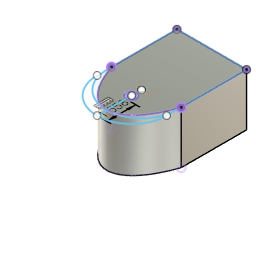
1759811952310_peo6bbk9y (Autodesk Fusion 360 archive; units mm, degrees)
design "dado_v3"
part number: 2025-08-25-22-53-08-385
Autodesk Fusion 360 part; units mm, degrees
sketch "Sketch1" plane through (0, 0, 0) normal (0, 0, 1) x (1, 0, 0)
  circle A0 centre (0, 0) radius 50.8
  line L0 (-50.8, 0) -> (50.8, 0)
  line L1 (50.8, 0) -> (50.8, 102.3291)
  line L2 (50.8, 102.3291) -> (-50.8, 102.3291)
  line L3 (-50.8, 102.3291) -> (-50.8, 0)
  dimension "d1" = 101.6
  constraint coincident A0.centre origin
  constraint horizontal L0
  constraint vertical L1
  constraint horizontal L2
  constraint vertical L3
  constraint coincident A0 L0.start
  constraint tangent A0 L1
  constraint tangent A0 L3
  measures "d1" diameter of A0
extrude "Extrude1" add sketch "Sketch1" along normal blind 76.2
sketch "Sketch2" plane through (0, 0, 76.2) normal (0, 0, 1) x (-1, 0, 0)
  line L0 (50.8, -102.3291) -> (50.8, 0)
  arc A0 (50.8, 0) -> (-50.8, 0) centre (0, 0) ccw
  line L1 (-50.8, 0) -> (-50.8, -102.3291)
  line L2 (-50.8, -102.3291) -> (50.8, -102.3291)
  circle A1 centre (-29.5656, 14.9606) radius 6.731
  circle A2 centre (-29.5656, -10.4394) radius 6.731
  circle A3 centre (-29.5656, -35.8394) radius 6.731
  circle A4 centre (29.5656, -35.8394) radius 6.731
  circle A5 centre (29.5656, -10.4394) radius 6.731
  circle A6 centre (29.5656, 14.9606) radius 6.731
  circle A7 centre (0, 14.9606) radius 7.874
  circle A8 centre (0, -35.8394) radius 7.874
  line L3 (0, 50.8) -> (0, 22.8346)
  line L4 (0, 14.9606) -> (-29.5656, 14.9606)
  line L5 (0, 14.9606) -> (29.5656, 14.9606)
  line L6 (-29.5656, -35.8394) -> (29.5656, -35.8394)
  line L7 (0, -35.8394) -> (0, -63.8048)
  dimension "d4" = 13.462
  dimension "d10" = 15.748
  dimension "d11" = 25.4
  dimension "d12" = 25.4
  dimension "d13" = 25.4
  dimension "d14" = 25.4
  dimension "d15" = 21.2344
  dimension "d16" = 21.2344
  dimension "d17" = 21.2344
  dimension "d18" = 21.2344
  dimension "d19" = 21.2344
  dimension "d20" = 21.2344
  dimension "d21" = 27.9654
  dimension "d22" = 27.9654
  constraint equal A1 A2
  constraint equal A1 A3
  constraint equal A1 A6
  constraint equal A1 A5
  constraint equal A1 A4
  constraint equal A7 A8
  constraint midpoint A0 L3.start
  constraint coincident A7 L3.end
  constraint vertical L3
  constraint coincident A7.centre L4.start
  constraint horizontal L4
  constraint coincident A1.centre L4.end
  constraint parallel L4 L5
  constraint coincident A6.centre L5.end
  constraint coincident A3.centre L6.start
  constraint coincident A4.centre L6.end
  constraint coincident A8.centre L6
  constraint coincident A8.centre L7.start
  constraint perpendicular L6 L7
  measures "d4" diameter of A1
  measures "d10" diameter of A7
  measures "d11" distance of A1.centre A2.centre
  measures "d12" distance of A2.centre A3.centre
  measures "d13" vertical distance of A5.centre A6.centre
  measures "d14" distance of A4.centre A5.centre
  measures "d15" distance of L1 A1.centre
  measures "d16" distance of L0 A6.centre
  measures "d17" distance of L1 A2.centre
  measures "d18" distance of L1 A3.centre
  measures "d19" distance of L0 A5.centre
  measures "d20" distance of L0 A4.centre
  measures "d21" distance of L3.start L3.end
  measures "d22" distance of A8.centre L7.end
extrude "Extrude2" cut sketch "Sketch2" against normal blind 101.6 contours A7 L4 L5 | A7 L4 L5
sketch "Sketch3" plane through (0, 0, 76.2) normal (0, 0, 1) x (-1, 0, 0)
  circle A0 centre (0, 14.9606) radius 7.874
  line L0 (50.8, -102.3291) -> (50.8, 0)
  arc A1 (50.8, 0) -> (-50.8, 0) centre (0, 0) ccw
  line L1 (-50.8, 0) -> (-50.8, -102.3291)
  line L2 (-50.8, -102.3291) -> (50.8, -102.3291)
  line L3 (-44.45, 12.7) -> (44.45, 12.7)
  line L4 (44.45, 12.7) -> (44.45, -102.3291)
  line L5 (44.45, -102.3291) -> (-44.45, -102.3291)
  line L6 (-44.45, -102.3291) -> (-44.45, 12.7)
  line L7 (0, 50.8) -> (0, 12.7)
  line L8 (0, 12.7) -> (0, 185.42)
  line L9 (-62.23, -56.8043) -> (62.23, -56.8043)
  spline S0 degree 2 poles (-62.23, -56.8043) (0, 395.5384) (62.23, -56.8043) knots 0 0 0 24.849245 24.849245 24.849245 weights 1 0.311883 1
  line L10 (-44.45, 9.235) -> (0, 9.235)
  line L11 (0, 50.8) -> (50.8, 50.8)
  line L12 (50.8, 50.8) -> (50.8, 0)
  line L13 (50.8, 0) -> (0, 0)
  line L14 (0, 0) -> (0, 50.8)
  line L15 (-43.815, 12.7) -> (43.815, 12.7)
  spline S1 degree 2 poles (43.815, 12.7) (0, 129.3943) (-43.815, 12.7) knots 0 0 0 12.094999 12.094999 12.094999 weights 1 0.555689 1
  line L16 (0, 12.7) -> (0, 17.78)
  dimension "d25" = 88.9
  dimension "d26" = 101.6
  dimension "d27" = 6.35
  dimension "d28" = 38.1
  dimension "d35" = 124.46
  dimension "d36" = 62.23
  dimension "d39" = 50.8
  constraint horizontal L3
  constraint vertical L4
  constraint horizontal L5
  constraint vertical L6
  constraint coincident L2 L4.end
  constraint midpoint A1 L7.start
  constraint perpendicular L3 L7
  constraint coincident L3 L7.end
  constraint perpendicular L3 L8
  constraint perpendicular L0 L9
  constraint coincident S0 L10.start
  constraint coincident L6 L10.start
  constraint perpendicular L6 L10
  constraint horizontal L11
  constraint vertical L12
  constraint horizontal L13
  constraint vertical L14
  constraint collinear L3 L15
  constraint midpoint L15 L7.end
  constraint perpendicular L15 L16
  constraint collinear L7 L16
  measures "d25" distance of L3.start L3.end
  measures "d26" distance of L0.start L1.end
  measures "d27" distance of L1 L6
  measures "d28" distance of L7.start L7.end
  measures "d35" distance of L9.start L9.end
  measures "d36" horizontal distance of L7.end L9.start
  measures "d39" distance of L7.start A1.centre
extrude "Extrude3" cut sketch "Sketch3" against normal blind 76.2 contours A1 L3 L7 L8 S0 L14 L15 S1 | A1 L3 L7 L8 S0 L14 L15 S1 | L3 L4 S0 L15 | L3 L6 S0 L15 | A1 L11 S1 | A1 L3 L4 S0 L13 S1 | A1 L1 L3 L6 S0 S1 | A1 L11 L12 S1 | L0 S0 L13
sketch "Sketch4" plane through (0, 0, 0) normal (0, 0, -1) x (1, 0, 0)
  line L0 (-50.8, -102.3291) -> (50.8, -102.3291)
  spline S0 degree 2 poles (50.8, -6.8994) (0, 142.0403) (-50.8, -6.8994) knots 4.267607 4.267607 4.267607 20.581638 20.581638 20.581638 weights 0.804237 0.507646 0.804237
  line L1 (-50.8, -6.8994) -> (-50.8, -102.3291)
  line L2 (50.8, -102.3291) -> (50.8, -6.8994)
  circle A0 centre (0, 14.9606) radius 7.874
sketch "Sketch5" plane through (0, 0, 0) normal (0, 0, -1) x (1, 0, 0)
  spline S0 degree 2 poles (50.8, -6.8994) (0, 142.0403) (-50.8, -6.8994) knots 4.267607 4.267607 4.267607 20.581638 20.581638 20.581638 weights 0.804237 0.507646 0.804237
sketch "Sketch7" plane through (0, 0, 76.2) normal (0, 0, 1) x (-1, 0, 0)
  circle A0 centre (0, 14.9606) radius 7.874
  line L0 (50.8, -102.3291) -> (50.8, -6.8994)
  line L1 (-50.8, -6.8994) -> (-50.8, -102.3291)
  line L2 (-50.8, -102.3291) -> (50.8, -102.3291)
  line L3 (-50.8, 0) -> (-50.8, -102.3291)
  circle A1 centre (0, 14.9606) radius 7.874
  line L4 (50.8, -102.3291) -> (50.8, 0)
  line L5 (-50.8, -102.3291) -> (50.8, -102.3291)
  arc A2 (50.8, 0) -> (-50.8, 0) centre (0, 0) ccw
  line L6 (0, 22.8346) -> (0, 64.9478)
  arc A3 (50.8, 14.1478) -> (-50.8, 14.1478) centre (0, 14.1478) ccw
  spline S0 degree 2 poles (50.8, -6.8994) (0, 142.0403) (-50.8, -6.8994) knots -20.581638 -20.581638 -20.581638 -4.267607 -4.267607 -4.267607 weights 0.804237 0.507646 0.804237
  spline S1 degree 2 poles (-50.8, -6.8994) (0, 142.0403) (50.8, -6.8994) knots 4.267607 4.267607 4.267607 20.581638 20.581638 20.581638 weights 0.804237 0.507646 0.804237
  dimension "d44" = 42.1132
  constraint coincident A1 L6.start
  constraint vertical L6
  measures "d44" distance of L6.start L6.end
equation "d12 = d11"
equation "d13 = d11"
equation "d14 = d11"
equation "d15 = 0.571 in + ( d4 / 2 )"
equation "d16 = d15"
equation "d17 = d15"
equation "d18 = d15"
equation "d19 = d16"
equation "d20 = d16"
equation "d27 = ( d26 - d25 ) / 2"
equation "d36 = d35 / 2"
